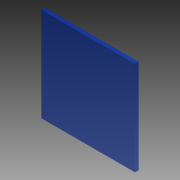
# Autodesk Inventor part: tray
Saved by Autodesk Inventor 2014 SP2 (Build 180246200, 246)
## iProperties
Created: 2016-09-18
Part Number: tray
Material: Generic
Document SubType Name: Modeling
Designer: cruiser
Density: 1 g/cm^3
Appearance: Default
Mass: 132.3 g
Surface Area: 485.28 cm^2
Volume: 132.3 cm^3
Author: cruiser
Autodesk Inventor part; units mm, degrees
ref_plane "YZ Plane" through (0, 0, 0) normal (1, 0, 0) x (0, 1, 0)
ref_plane "XZ Plane" through (0, 0, 0) normal (0, 1, 0) x (-1, 0, 0)
ref_plane "XY Plane" through (0, 0, 0) normal (0, 0, 1) x (1, 0, 0)
sketch "Sketch1" plane through (0, 0, 0) normal (0, 1, 0) x (-1, 0, 0)
  line L0 (-75, -75) -> (75, -75)
  line L1 (75, -75) -> (75, 75)
  line L2 (75, 75) -> (-75, 75)
  line L3 (-75, 75) -> (-75, -75)
  line L4 (-75, -75) -> (75, 75) construction
  line L5 (75, -75) -> (-75, 75) construction
  point P0 (0, 0)
  dimension "d0" = 150
  dimension "d1" = 150
  constraints: 12 end point, 2 midpoint, 2 parallel, 1 horizontal, 1 perpendicular
  measures "d0" distance of L2.end L1.end
  measures "d1" distance of L1.end L0.end
extrude "Extrusion1" add sketch "Sketch1" along normal blind 5.88
equation "\"d0\" = tray_x"
equation "\"d1\" = tray_y"
equation "\"d2\" = tray_t"
equation "\"laserresin\" = 5"
equation "\"st1_thickness\" = 1.5875"
equation "\"st2_thickness\" = 1.5875"
equation "\"st3_thickness\" = 1.5875"
equation "\"al1_thickness\" = 1.5875"
equation "\"al2_thickness\" = 1.5875"
equation "\"al3_thickness\" = 1.5875"
equation "\"bend_factor\" = 2.26205"
equation "\"st1_bend\" = 3.591"
equation "\"st2_bend\" = 3.591"
equation "\"st3_bend\" = 3.591"
equation "\"al1_bend\" = 3.591"
equation "\"al2_bend\" = 3.591"
equation "\"al3_bend\" = 3.591"
equation "\"acrylic1_thickness\" = 5.88"
equation "\"acrylic2_thickness\" = 3.15"
equation "\"acrylic3_thickness\" = 3.15"
equation "\"nema17_l\" = 48"
equation "\"nema17_x\" = 43"
equation "\"switch_spacing\" = 19"
equation "\"laser_body_diameter\" = 12"
equation "\"m3_diameter\" = 3"
equation "\"m3_head\" = 6"
equation "\"m4_diameter\" = 4"
equation "\"m5_diameter\" = 5"
equation "\"m5_head\" = 10.3"
equation "\"rivet_diameter\" = 3.3"
equation "\"brass_insert_drill\" = 4"
equation "\"m5_brass_insert_drill\" = 6.7"
equation "\"m3_press_nut_drill\" = 4.5"
equation "\"m5_press_nut_drill\" = 6.5"
equation "\"linear_bearing_spacing\" = 198"
equation "\"platform_t\" = 1.5875"
equation "\"platform_fold_x\" = 25"
equation "\"platform_crane_gap\" = 0.1"
equation "\"platform_upper_y\" = 46.625"
equation "\"crane_t\" = 1.5875"
equation "\"crane_x\" = 223"
equation "\"crane_gap\" = 0.1"
equation "\"crane_z\" = 48"
equation "\"tray_t\" = 5.88"
equation "\"tray_x\" = 150"
equation "\"tray_y\" = 150"
equation "\"reservoir_t\" = 1.5875"
equation "\"frame_front_t\" = 1.5875"
equation "\"frame_gap\" = 0.1"
equation "\"frame_back_t\" = 1.5875"
equation "\"frame_back_x\" = 266.625"
equation "\"frame_back_y\" = 66.625"
equation "\"frame_back_z\" = 496.625"
equation "\"drawer_t\" = 1.5875"
equation "\"drawer_x\" = 193.375"
equation "\"drawer_y\" = 65"
equation "\"dawer_top_y\" = 0"
equation "\"drawer_fold\" = 15"
equation "\"foot_t\" = 1.5875"
equation "\"foot_x\" = 193.375"
equation "\"foot_z\" = 15"
equation "\"nema17_shaft\" = 24"
equation "\"drawer_window_gap\" = 5"
equation "\"reservoir_flap_y\" = 21.5875"
equation "\"drawer_gap\" = 0.1"
equation "\"tray_to_platform_oversize\" = 0"
equation "\"lmk8uu_shaft\" = 15"
equation "\"lmk8uu_x\" = 25"
equation "\"lmk8uu_z\" = 24"
equation "\"drawer_reservoir_overlap_x\" = 18.4125"
equation "\"frame_front_fold\" = 15"
body "Solid1"
